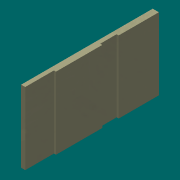
# Autodesk Inventor part: leftSide
Saved by Autodesk Inventor 2016 (Build 200138000, 138)
## iProperties
Created: 2015-10-13
Part Number: leftSide
Material: PC/ABS Plastic
Document SubType Name: Modeling
Designer: Sawaiz
Density: 0.357273 g/cm^3
Appearance: Smooth - Ash
Author: Sawaiz
Autodesk Inventor part; units mm, degrees
ref_plane "YZ Plane" through (0, 0, 0) normal (1, 0, 0) x (0, 1, 0)
ref_plane "XZ Plane" through (0, 0, 0) normal (0, 1, 0) x (-1, 0, 0)
ref_plane "XY Plane" through (0, 0, 0) normal (0, 0, 1) x (1, 0, 0)
sketch "Sketch1" plane through (0, 0, 0) normal (0, 1, 0) x (-1, 0, 0)
  line L0 (-101.6, 55.5625) -> (101.6, 55.5625)
  line L1 (101.6, 55.5625) -> (101.6, -55.5625)
  line L2 (101.6, -55.5625) -> (-101.6, -55.5625)
  line L3 (-101.6, -55.5625) -> (-101.6, 55.5625)
  line L4 (-101.6, 55.5625) -> (101.6, -55.5625) construction
  line L5 (101.6, 55.5625) -> (-101.6, -55.5625) construction
  point P0 (0, 0)
  dimension "d0" = 203.2
  dimension "d1" = 111.125
  constraints: 12 end point, 2 midpoint, 2 parallel, 1 horizontal, 1 perpendicular
  measures "d0" distance of L1.end L2.end
  measures "d1" distance of L0.end L1.end
extrude "Extrusion1" add sketch "Sketch1" along normal blind 9.525
sketch "Sketch8" plane through (0, 9.525, 0) normal (0, 1, 0) x (1, 0, 0)
  line L0 (-101.6, -55.5625) -> (101.6, -55.5625) projected
  line L1 (101.6, -55.5625) -> (101.6, 55.5625) projected
  line L2 (101.6, 55.5625) -> (-101.6, 55.5625) projected
  line L3 (-101.6, 55.5625) -> (-101.6, -55.5625) projected
  line L4 (101.6, 55.5625) -> (-101.6, 55.5625) projected
  line L5 (101.6, -55.5625) -> (57.276, -55.5625)
  line L6 (57.276, -55.5625) -> (57.276, 55.5625)
  line L7 (57.276, 55.5625) -> (101.6, 55.5625)
  line L8 (101.6, 55.5625) -> (101.6, -55.5625)
  line L9 (-14.1615, -55.5625) -> (-39.5615, -55.5625)
  line L10 (-39.5615, -55.5625) -> (-39.5615, 55.5625)
  line L11 (-39.5615, 55.5625) -> (-14.1615, 55.5625)
  line L12 (-14.1615, 55.5625) -> (-14.1615, -55.5625)
  point P0 (0, 0)
  dimension "d40" = 44.324
  dimension "d41" = 25.4
  dimension "d44" = 71.4375
  constraints: 16 end point, 4 parallel, 4 point on line, 2 horizontal, 2 perpendicular, 1 collinear
  measures "d40" distance between parallel lines of L1 L6
  measures "d41" distance between parallel lines of L10 L12
  measures "d44" distance between parallel lines of L6 L12
extrude "Extrusion5" cut sketch "Sketch8" against normal blind 3.175 contours L10 L2 L12 L0 | L6 L2 L1 L0
equation "\"d0\" = depth"
equation "\"d1\" = height + 1.5 * internalAcrylicThickness"
equation "\"d2\" = acrylicThickness"
equation "\"d40\" = centerThickness + aerogelThickness + 2 * internalAcrylicThickness + fresnelThickness"
equation "\"d41\" = internalAcrylicThickness + sensorHolderDepth"
equation "\"d42\" = 0.5 * internalAcrylicThickness"
equation "\"acrylicThickness\" = 9.525"
equation "\"depth\" = 203.2"
equation "\"mirrorThickness\" = 3.175"
equation "\"height\" = 101.6"
equation "\"width\" = 101.6"
equation "\"mirrorAngle\" = 5deg"
equation "\"detectorWidth\" = 52"
equation "\"detectorHeight\" = 52"
equation "\"fresnelThickness\" = 0.1"
equation "\"focalLength\" = 76.2"
equation "\"ior\" = 1.49"
equation "\"centerThickness\" = 1.524"
equation "\"fresnelAngle\" = 90deg"
equation "\"fresnelEffectiveDiameter\" = 76.2"
equation "\"mirrorSuppourtWidth\" = 38.1"
equation "\"backGrooveBit\" = 4.8006"
equation "\"sensorHolderSensorWidth\" = 53.975"
equation "\"sensorHolderWidth\" = 88.9"
equation "\"sensorHolderSesnorHeight\" = 53.975"
equation "\"sensorHolderHeight\" = 88.9"
equation "\"sensorHolderSensorHeight\" = 53.975"
equation "\"sensorHolderORingGroove\" = 3.175"
equation "\"sensorHolderORing\" = 3.175"
equation "\"sensorHolderFlushORingID\" = 304.8"
equation "\"sensorHolderFlushORing\" = 3.175"
equation "\"frontBackORingID\" = 419.1"
equation "\"oRingWidth\" = 1.5875"
equation "\"sensorHolderORingID\" = 203.2"
equation "\"topBottomHorizontalMirrorGroove\" = 12.7"
equation "\"backMirrorGroove\" = 6.35"
equation "\"mirrorGroove\" = 19.05"
equation "\"fresnelChamfer\" = 6.35"
equation "\"mirrorGrooveFillet\" = 6.35"
equation "\"mirrorGrooveDrill\" = 6.35"
equation "\"mirrorGrooveMill\" = 3.175"
equation "\"fresnelMirrorChamfer\" = 6.35"
equation "\"detectorOpeningHeight\" = 76.2"
equation "\"detectorOpeningWidth\" = 76.2"
equation "\"sensorHolderDepth\" = 19.05"
equation "\"internalAcrylicThicnkess\" = 6.35"
equation "\"frameAcrylicThickness\" = 9.525"
equation "\"aerogelHeight\" = 101.6"
equation "\"aerogelWidth\" = 101.6"
equation "\"internalAcrylicThickness\" = 6.35"
equation "\"aerogelThickness\" = 30"
body "Solid1"
